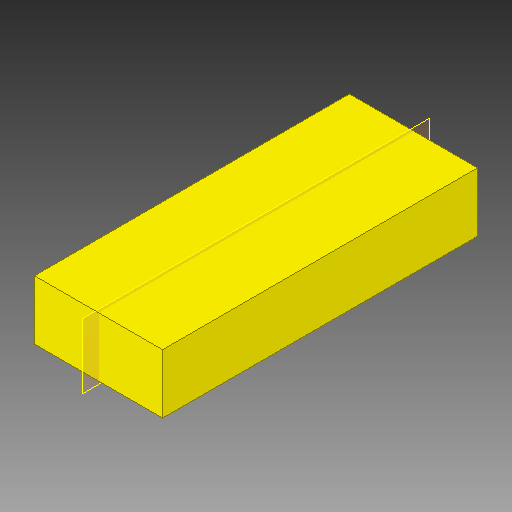
# Autodesk Inventor part: Battery_37v_320mAh
Saved by Autodesk Inventor 2019.4 (Build 234330000, 330)
## iProperties
Created: 2021-06-27
Part Number: Battery_37v_320mAh
Material: Generic
Document SubType Name: Modeling
Designer: keshav
Density: 1 g/cm^3
Appearance: Default
Author: keshav
Autodesk Inventor part; units mm, degrees
ref_plane "XZ Plane" through (0, 0, 0) normal (0, 1, 0) x (-1, 0, 0)
ref_plane "XY Plane" through (0, 0, 0) normal (0, 0, 1) x (1, 0, 0)
sketch "Sketch1" plane through (0, 0, 0) normal (0, 1, 0) x (-1, 0, 0)
  line L0 (-7.575, 18.625) -> (7.575, 18.625)
  line L1 (7.575, 18.625) -> (7.575, -18.625)
  line L2 (7.575, -18.625) -> (-7.575, -18.625)
  line L3 (-7.575, -18.625) -> (-7.575, 18.625)
  line L4 (-7.575, 18.625) -> (7.575, -18.625) construction
  line L5 (7.575, 18.625) -> (-7.575, -18.625) construction
  point P0 (0, 0)
  dimension "d0" = 15.15
  dimension "d1" = 37.25
  constraints: 12 end point, 2 midpoint, 2 parallel, 1 horizontal, 1 perpendicular
  measures "d0" distance of L1.end L2.end
  measures "d1" distance of L0.end L1.end
extrude "Extrusion1" add sketch "Sketch1" along normal blind 7
body "Solid1"
